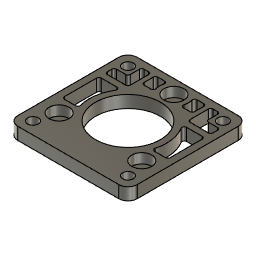
Laser Shroud Magnetic Mount (Autodesk Fusion 360 design; units mm, degrees)
Autodesk Fusion 360 part; units mm, degrees
sketch "Sketch1" plane through (0, 0, 0) normal (0, 0, 1) x (1, 0, 0) in component "Laser Shroud Mount"
  line L0 (0, 0) -> (39, 0)
  line L1 (39, 0) -> (39, 39)
  line L2 (39, 39) -> (0, 39)
  line L3 (0, 39) -> (0, 0)
  dimension "d1" = 39
  dimension "d2" = 39
  constraint horizontal L0
  constraint vertical L1
  constraint horizontal L2
  constraint vertical L3
  constraint coincident L0.start L3.end
  measures "d1" distance of L0.start L0.end
  measures "d2" distance of L0.start L2.end
extrude "Extrude1" add sketch "Sketch1" along normal blind 4 in component "Laser Shroud Mount"
sketch "Sketch2" plane through (0, 0, 4) normal (0, 0, 1) x (-1, 0, 0) in component "Laser Shroud Mount"
  line L0 (0, -39) -> (0, 0)
  line L1 (0, 0) -> (-39, 0)
  line L2 (-39, 0) -> (-39, -39)
  line L3 (-39, -39) -> (0, -39)
  line L4 (-19.5, -39) -> (-19.5, 0) construction
  line L5 (0, -19.5) -> (-39, -19.5) construction
  circle A0 centre (-19.5, -19.5) radius 10.6
  line L6 (-35, -35) -> (-4, -35) construction
  line L7 (-4, -35) -> (-4, -4) construction
  line L8 (-4, -4) -> (-35, -4) construction
  line L9 (-35, -4) -> (-35, -35) construction
  line L10 (-35, -35) -> (-4, -4) construction
  line L11 (-4, -35) -> (-35, -4) construction
  circle A1 centre (-4, -35) radius 1.75
  circle A2 centre (-35, -35) radius 1.75
  circle A3 centre (-4, -4) radius 1.75
  circle A4 centre (-35, -4) radius 1.75
  point P0 (-19.5, -19.5)
  dimension "d5" = 21.2
  dimension "d6" = 31
  dimension "d7" = 31
  dimension "d8" = 3.5
  dimension "d9" = 3.5
  dimension "d10" = 3.5
  dimension "d11" = 3.5
  constraint midpoint L3 L4.start
  constraint midpoint L1 L4.end
  constraint midpoint L0 L5.start
  constraint midpoint L2 L5.end
  constraint midpoint L5 P0
  constraint horizontal L6
  constraint perpendicular L6 L7
  constraint parallel L6 L8
  constraint parallel L7 L9
  constraint coincident L10 P0
  constraint coincident L11 P0
  constraint coincident P0 A0.centre
  constraint coincident L6.end L7.start
  constraint coincident L6.start L9.end
  constraint coincident L7.end L8.start
  constraint coincident L8.end L9.start
  measures "d5" diameter of A0
  measures "d6" distance of L7.end L8.end
  measures "d7" distance of L6.end L7.end
  measures "d8" diameter of A1
  measures "d9" diameter of A2
  measures "d10" diameter of A3
  measures "d11" diameter of A4
extrude "Extrude2" cut sketch "Sketch2" against normal up to surface (4 mm away) contours A0 | A1 | A2 | A3 | A4 in component "Laser Shroud Mount"
sketch "Sketch3" plane through (0, 0, 4) normal (0, 0, 1) x (-1, 0, 0) in component "Laser Shroud Mount"
  circle A0 centre (-4, -35) radius 1.75
  circle A1 centre (-19.5, -19.5) radius 10.6
  circle A2 centre (-35, -35) radius 1.75
  circle A3 centre (-4, -4) radius 1.75
  circle A4 centre (-35, -4) radius 1.75
  line L0 (0, -39) -> (0, 0)
  line L1 (0, 0) -> (-39, 0)
  line L2 (-39, 0) -> (-39, -39)
  line L3 (-39, -39) -> (0, -39)
  line L4 (-19.5, -39) -> (-19.5, 0) construction
  line L5 (0, -34.5) -> (-39, -34.5) construction
  circle A5 centre (-19.5, -34.5) radius 3.25
  line L6 (0, -10.5) -> (-39, -10.5) construction
  line L7 (-6, -39) -> (-6, 0) construction
  circle A6 centre (-6, -10.5) radius 3.25
  line L8 (-33, -39) -> (-33, 0) construction
  circle A7 centre (-33, -10.5) radius 3.25
  dimension "d14" = 4.5
  dimension "d15" = 6.5
  dimension "d16" = 6.5
  dimension "d18" = 10.5
  dimension "d19" = 6
  dimension "d21" = 6
  dimension "d22" = 6.5
  constraint midpoint L3 L4.start
  constraint midpoint L1 L4.end
  constraint coincident L0 L5.start
  constraint coincident L2 L5.end
  constraint perpendicular L2 L5
  constraint midpoint L5 A5.centre
  constraint coincident L0 L6.start
  constraint coincident L2 L6.end
  constraint perpendicular L2 L6
  constraint coincident L1 L7.end
  constraint perpendicular L1 L7
  constraint coincident L7 A6.centre
  constraint coincident L6 A6.centre
  constraint coincident L3 L8.start
  constraint coincident L1 L8.end
  constraint perpendicular L1 L8
  constraint coincident L8 A7.centre
  constraint coincident L6 A7.centre
  measures "d14" distance of L3 L5
  measures "d15" diameter of A5
  measures "d16" diameter of A6
  measures "d18" distance of L1 L6
  measures "d19" distance of L0 L7
  measures "d21" distance of L2 L8
  measures "d22" diameter of A7
extrude "Extrude3" cut sketch "Sketch3" against normal blind 3.2 contours A5 | A6 | A7 in component "Laser Shroud Mount"
sketch "Sketch4" plane through (0, 0, 4) normal (0, 0, 1) x (-1, 0, 0) in component "Laser Shroud Mount"
  circle A0 centre (-19.5, -34.5) radius 3.25 construction
  circle A1 centre (-6, -10.5) radius 3.25
  circle A2 centre (-33, -10.5) radius 3.25
  circle A3 centre (-4, -35) radius 1.75
  circle A4 centre (-19.5, -19.5) radius 10.6
  circle A5 centre (-35, -35) radius 1.75
  circle A6 centre (-4, -4) radius 1.75
  circle A7 centre (-35, -4) radius 1.75
  line L0 (0, -39) -> (0, 0)
  line L1 (0, 0) -> (-39, 0)
  line L2 (-39, 0) -> (-39, -39)
  line L3 (-39, -39) -> (0, -39)
  line L4 (0, -36.75) -> (-39, -36.75) construction
  line L5 (-6.75, -39) -> (-6.75, 0) construction
  line L6 (-32.25, -39) -> (-32.25, 0) construction
  line L7 (0, -32.25) -> (-39, -32.25) construction
  line L8 (-6.75, -36.75) -> (-6.75, -32.25)
  line L9 (-2.25, -39) -> (-2.25, 0) construction
  line L10 (-6.75, -32.25) -> (-2.25, -32.25)
  line L11 (-2.25, -32.25) -> (-2.25, -29.25)
  line L12 (0, -19.5) -> (-39, -19.5) construction
  line L13 (-19.5, -39) -> (-19.5, 0) construction
  line L14 (-6.75, -36.75) -> (-9.75, -36.75)
  line L15 (-2.25, -29.25) -> (-9.75, -29.25)
  line L16 (-9.75, -29.25) -> (-9.75, -36.75)
  line L17 (-11.25, -36.75) -> (-11.25, -32.25)
  line L18 (-11.25, -36.75) -> (-15.3167, -36.75)
  line L19 (-11.25, -32.25) -> (-15.3167, -32.25)
  line L20 (-2.25, -27.25) -> (-9.5653, -27.25)
  line L21 (-2.25, -15.25) -> (-7.6384, -15.25)
  line L22 (-2.25, -27.25) -> (-2.25, -15.25)
  line L23 (0, -2) -> (-39, -2) construction
  arc A8 (-9.5653, -27.25) -> (-7.6384, -15.25) centre (-19.5, -19.5) ccw
  arc A9 (-15.3167, -36.75) -> (-15.3167, -32.25) centre (-19.5, -34.5) ccw
  arc A10 (-31.3616, -15.25) -> (-29.4347, -27.25) centre (-19.5, -19.5) ccw
  line L24 (-36.75, -15.25) -> (-31.3616, -15.25)
  line L25 (-36.75, -27.25) -> (-36.75, -15.25)
  line L26 (-36.75, -27.25) -> (-29.4347, -27.25)
  line L27 (-36.75, -29.25) -> (-29.25, -29.25)
  line L28 (-36.75, -32.25) -> (-36.75, -29.25)
  line L29 (-29.25, -29.25) -> (-29.25, -36.75)
  line L30 (-32.25, -32.25) -> (-36.75, -32.25)
  line L31 (-32.25, -36.75) -> (-32.25, -32.25)
  line L32 (-32.25, -36.75) -> (-29.25, -36.75)
  line L33 (-27.75, -36.75) -> (-27.75, -32.25)
  arc A11 (-23.6833, -32.25) -> (-23.6833, -36.75) centre (-19.5, -34.5) ccw
  line L34 (-27.75, -32.25) -> (-23.6833, -32.25)
  line L35 (-27.75, -36.75) -> (-23.6833, -36.75)
  dimension "d25" = 2.25
  dimension "d26" = 6.75
  dimension "d27" = 6.75
  dimension "d28" = 6.75
  dimension "d29" = 3
  dimension "d34" = 3
  dimension "d35" = 1.5
  dimension "d36" = 2
  dimension "d37" = 12
  dimension "d38" = 2
  constraint coincident L0 L4.start
  constraint coincident L2 L4.end
  constraint perpendicular L2 L4
  constraint coincident L3 L5.start
  constraint coincident L1 L5.end
  constraint perpendicular L1 L5
  constraint coincident L3 L6.start
  constraint coincident L1 L6.end
  constraint perpendicular L1 L6
  constraint coincident L0 L7.start
  constraint coincident L2 L7.end
  constraint perpendicular L2 L7
  constraint coincident L4 L8.start
  constraint coincident L5 L8.start
  constraint coincident L5 L8.end
  constraint coincident L7 L8.end
  constraint perpendicular L7 L8
  constraint coincident L3 L9.start
  constraint coincident L1 L9.end
  constraint perpendicular L1 L9
  constraint tangent A3 L9
  constraint coincident L9 L10.end
  constraint coincident L7 L10.end
  constraint perpendicular L7 L11
  constraint midpoint L0 L12.start
  constraint midpoint L2 L12.end
  constraint midpoint L3 L13.start
  constraint midpoint L1 L13.end
  constraint perpendicular L8 L14
  constraint perpendicular L11 L15
  constraint perpendicular L4 L16
  constraint coincident L4 L17.start
  constraint coincident L7 L17.end
  constraint perpendicular L7 L17
  constraint coincident L4 L18.end
  constraint coincident L7 L19.end
  constraint coincident L9 L20.start
  constraint perpendicular L9 L20
  constraint coincident L9 L21.start
  constraint perpendicular L5 L21
  constraint coincident L0 L23.start
  constraint coincident L2 L23.end
  constraint perpendicular L2 L23
  constraint concentric A4 A8
  constraint symmetric L8.start L13 L31.start
  constraint symmetric L8.end L13 L30.start
  constraint symmetric L10.end L13 L28.start
  constraint symmetric L11.end L13 L27.start
  constraint symmetric L13 L14.end L29.end
  constraint symmetric L13 L15.end L27.end
  constraint symmetric L13 L17.start L33.start
  constraint symmetric L13 L17.end L33.end
  constraint symmetric L13 L18.end A11.end
  constraint symmetric L13 L19.end A11.start
  constraint symmetric L13 L20.start L25.start
  constraint symmetric L13 L20.end A10.end
  constraint symmetric L13 L21.start L24.start
  constraint symmetric L13 L21.end A10.start
  constraint symmetric L13 A8 A10
  constraint symmetric L13 A9 A11
  measures "d25" distance of L3 L4
  measures "d26" distance of L0 L5
  measures "d27" distance of L2 L6
  measures "d28" distance of L3 L7
  measures "d29" distance of L10.end L11.end
  measures "d34" distance of L8.start L14.end
  measures "d35" distance of L16 L17
  measures "d36" distance of L15 L20
  measures "d37" distance of L20 L21
  measures "d38" distance of L1 L23
extrude "Extrude4" cut sketch "Sketch4" against normal up to surface (4 mm away) contours L8 L10 L11 L14 L15 L16 | L17 L18 L19 A9 | L20 L21 L22 A8 | A10 L24 L25 L26 | L27 L28 L29 L30 L31 L32 | L33 A11 L34 L35 in component "Laser Shroud Mount"
fillet "Fillet1" radius 3 4 edges at (0, 39, 2) (0, 0, 2) (39, 0, 2) (39, 39, 2) in component "Laser Shroud Mount"
fillet "Fillet3" radius 0.75 4 edges at (11.25, 36.75, 2) (11.25, 32.25, 2) (15.3167, 32.25, 2) (15.3167, 36.75, 2) in component "Laser Shroud Mount"
fillet "Fillet3" radius 0.75 4 edges at (23.6833, 36.75, 2) (23.6833, 32.25, 2) (27.75, 36.75, 2) (27.75, 32.25, 2) in component "Laser Shroud Mount"
fillet "Fillet3" radius 0.75 6 edges at (29.25, 36.75, 2) (32.25, 36.75, 2) (32.25, 32.25, 2) (36.75, 32.25, 2) (36.75, 29.25, 2) (29.25, 29.25, 2) in component "Laser Shroud Mount"
fillet "Fillet3" radius 0.75 6 edges at (6.75, 36.75, 2) (6.75, 32.25, 2) (2.25, 32.25, 2) (2.25, 29.25, 2) (9.75, 29.25, 2) (9.75, 36.75, 2) in component "Laser Shroud Mount"
fillet "Fillet3" radius 0.75 4 edges at (29.4347, 27.25, 2) (36.75, 27.25, 2) (36.75, 15.25, 2) (31.3616, 15.25, 2) in component "Laser Shroud Mount"
fillet "Fillet3" radius 0.75 4 edges at (2.25, 27.25, 2) (9.5653, 27.25, 2) (7.6384, 15.25, 2) (2.25, 15.25, 2) in component "Laser Shroud Mount"
component "Laser Shroud Mount" placed x (1, 0, 0) y (0, 1, 0) z (0, 0, 1) at (0, 0, 0)
